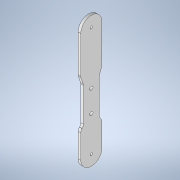
# Autodesk Inventor part: Brazo2Izquierda
Saved by Autodesk Inventor 2022 (Build 260153000, 153)
## iProperties
Created: 2021-09-13
Part Number: Brazo2Izquierda
Material: Generic
Document SubType Name: Modeling
Designer: Administrador
Density: 1 g/cm^3
Appearance: Default
Author: Administrador
Autodesk Inventor part; units mm, degrees
ref_plane "YZ Plane" through (0, 0, 0) normal (1, 0, 0) x (0, 1, 0)
ref_plane "XZ Plane" through (0, 0, 0) normal (0, 1, 0) x (-1, 0, 0)
ref_plane "XY Plane" through (0, 0, 0) normal (0, 0, 1) x (1, 0, 0)
sketch "Sketch1" plane through (0, 0, 0) normal (1, 0, 0) x (0, 1, 0)
  arc A0 (148.6113, 101.037) -> (148.6113, 125.037) centre (148.6113, 113.037) ccw
  circle A1 centre (88.6113, 113.037) radius 2
  line L0 (104.6113, 113.037) -> (96.6113, 113.037) construction
  line L1 (96.6113, 113.037) -> (96.6113, 122.037) construction
  line L2 (96.6113, 113.037) -> (96.6113, 104.037) construction
  line L3 (104.8415, 124.7804) -> (97.3811, 122.2936)
  line L4 (103.7624, 101.3554) -> (97.4602, 103.7186)
  line L5 (148.6113, 101.037) -> (105.518, 101.037)
  line L6 (148.6113, 125.037) -> (106.4227, 125.037)
  arc A2 (23.6113, 125.037) -> (23.6113, 101.037) centre (23.6113, 113.037) ccw
  line L7 (23.6113, 101.037) -> (49.9446, 101.037)
  line L8 (23.6113, 125.037) -> (50.5402, 125.037)
  circle A3 centre (23.6113, 113.037) radius 1.5
  circle A4 centre (63.6113, 113.037) radius 2
  line L9 (52.9446, 102.037) -> (54.278, 103.037)
  line L10 (54.0758, 123.5725) -> (54.1468, 123.5015)
  line L11 (47.6113, 113.037) -> (55.6113, 113.037) construction
  line L12 (55.6113, 113.037) -> (55.6113, 104.037) construction
  line L13 (55.6113, 113.037) -> (55.6113, 122.037) construction
  line L14 (76.1113, 122.037) -> (76.1113, 104.037) construction
  line L15 (57.278, 104.037) -> (95.7046, 104.037)
  line L16 (57.6824, 122.037) -> (95.7999, 122.037)
  arc A5 (54.0758, 123.5725) -> (50.5402, 125.037) centre (50.5402, 120.037) ccw
  arc A6 (57.278, 104.037) -> (54.278, 103.037) centre (57.278, 99.037) ccw
  arc A7 (49.9446, 101.037) -> (52.9446, 102.037) centre (49.9446, 106.037) ccw
  arc A8 (97.4602, 103.7186) -> (95.7046, 104.037) centre (95.7046, 99.037) ccw
  arc A9 (103.7624, 101.3554) -> (105.518, 101.037) centre (105.518, 106.037) ccw
  arc A10 (54.1468, 123.5015) -> (57.6824, 122.037) centre (57.6824, 127.037) ccw
  arc A11 (95.7999, 122.037) -> (97.3811, 122.2936) centre (95.7999, 127.037) ccw
  arc A12 (106.4227, 125.037) -> (104.8415, 124.7804) centre (106.4227, 120.037) ccw
  circle A13 centre (148.6113, 113.037) radius 1.5
  point P0 (1.5, 26.1095)
  point P1 (22.5, 26.1095)
  point P2 (1.5, 26.1095)
  point P3 (22.5, 26.1095)
  dimension "d44" = 4
  dimension "d46" = 8
  dimension "d47" = 9
  dimension "d48" = 9
  dimension "d50" = 8
  dimension "d53" = 24
  dimension "d54" = 3
  dimension "d57" = 4
  dimension "d59" = 8
  dimension "d60" = 9
  dimension "d61" = 9
  dimension "d63" = 8
  dimension "d64" = 40
  dimension "d65" = 25
  dimension "d100" = 5
  dimension "d102" = 3
  constraints: 34 end point, 20 point on circle, 18 tangent, 14 centre point, 8 point on line, 7 equal radius, 2 coincident, 2 perpendicular, 1 horizontal, 1 parallel
  measures "d44" diameter of A1
  measures "d46" distance of L0.start L2.start
  measures "d47" distance of L2.start L1.end
  measures "d48" distance of L2.start L2.end
  measures "d50" distance of A1.centre L2.start
  measures "d53" diameter of A2
  measures "d54" diameter of A3
  measures "d57" diameter of A4
  measures "d59" distance of L11.start L13.start
  measures "d60" distance of L13.start L12.end
  measures "d61" distance of L13.start L13.end
  measures "d63" distance of A4.centre L13.start
  measures "d64" distance of A2.centre A4.centre
  measures "d65" distance of A1.centre A4.centre
  measures "d100" radius of A5
  measures "d102" diameter of A13
extrude "Extrusion1" add sketch "Sketch1" along normal blind 3
body "Solid1"
